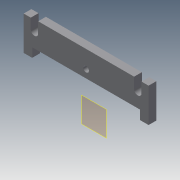
# Autodesk Inventor part: Upper Support
Saved by Autodesk Inventor 2014 SP1 (Build 180222100, 222)
## iProperties
Created: 2014-04-09
Part Number: Upper Support
Material: Generic
Document SubType Name: Modeling
Designer: tom
Density: 1 g/cm^3
Appearance: Default
Author: tom
Autodesk Inventor part; units mm, degrees
ref_plane "YZ Plane" through (0, 0, 0) normal (1, 0, 0) x (0, 1, 0)
ref_plane "XZ Plane" through (0, 0, 0) normal (0, 1, 0) x (-1, 0, 0)
ref_plane "XY Plane" through (0, 0, 0) normal (0, 0, 1) x (1, 0, 0)
ref_plane "Work Plane1" through (257.0292, -52.0592, 297.998) normal (0, 0, 1) x (1, 0, 0)
sketch "Sketch1" plane through (257.0292, -52.0592, 297.998) normal (0, 0, 1) x (1, 0, 0)
  line L0 (69.85, 69.215) -> (69.85, 31.115)
  line L1 (-69.85, 31.115) -> (-69.85, 69.215)
  arc A0 (-61.9125, 57.785) -> (-53.6575, 57.785) centre (-57.785, 57.785) ccw
  line L2 (-61.9125, 57.785) -> (-61.9125, 69.215)
  line L3 (-53.6575, 57.785) -> (-53.6575, 69.215)
  line L4 (-69.85, 69.215) -> (-61.9125, 69.215)
  line L5 (0, 69.215) -> (0, 28.575) construction
  arc A1 (53.6575, 57.785) -> (61.9125, 57.785) centre (57.785, 57.785) ccw
  line L6 (61.9125, 57.785) -> (61.9125, 69.215)
  line L7 (53.6575, 57.785) -> (53.6575, 69.215)
  line L8 (-53.6575, 69.215) -> (53.6575, 69.215)
  line L9 (61.9125, 69.215) -> (69.85, 69.215)
  line L10 (-60.325, 31.115) -> (-60.325, 41.275)
  line L11 (-60.325, 41.275) -> (60.325, 41.275)
  line L12 (60.325, 41.275) -> (60.325, 31.115)
  line L13 (69.85, 31.115) -> (60.325, 31.115)
  line L14 (-60.325, 31.115) -> (-69.85, 31.115)
  circle A2 centre (0, 50.275) radius 3.175
  point P0 (0, 0)
  dimension "d0" = 139.7
  dimension "d1" = 69.85
  dimension "d3" = 38.1
  dimension "d6" = 8.255
  dimension "d10" = 12.065
  dimension "d12" = 10.16
  dimension "d15" = 120.65
  dimension "d17" = 60.325
  dimension "d18" = 69.85
  dimension "d19" = 31.115
  dimension "d20" = 31.115
  dimension "d22" = 6.35
  dimension "d23" = 57.785
  dimension "d24" = 27.94
  constraints: 30 end point, 13 perpendicular, 7 parallel, 5 symmetric about line, 4 point on circle, 3 centre point, 3 horizontal, 2 tangent, 1 midpoint, 2 other
  measures "d0" distance of L0.end L1.start
  measures "d1" distance from line of point (0, 0) L0
  measures "d3" distance of L1.start L1.end
  measures "d6" diameter of A0
  measures "d10" distance from line of L1 A0.centre
  measures "d12" distance of L10.start L10.end
  measures "d15" distance of L10.end L11.end
  measures "d17" distance between parallel lines of L10 L5
  measures "d18" distance between parallel lines of L5 L1
  measures "d19" distance from line of point (0, 0) L14
  measures "d20" distance from line of point (0, 0) L13
  measures "d22" diameter of A2
  measures "d23" horizontal distance of point (0, 0) A0.centre
  measures "d24" distance between parallel lines of L11 L8
extrude "Extrusion1" add sketch "Sketch1" along normal blind 8.66
equation "\"d17\" = 0.5 * d15"
equation "\"d18\" = 0.5 * d0"
body "Solid1"
